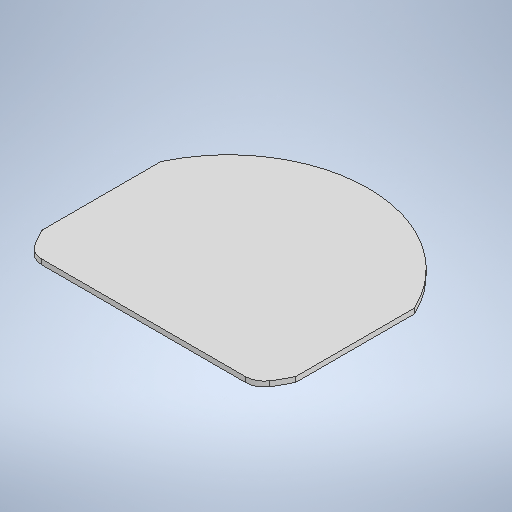
# Autodesk Inventor part: tapa_carcasa_4.0
Saved by Autodesk Inventor 2025.3 (Build 293356030, 356C)
## iProperties
Created: 2025-10-09
Part Number: tapa_carcasa_4.0
Material: Generic
Document SubType Name: Modeling
Designer: brene
Density: 1 g/cm^3
Appearance: Default
Author: brene
Autodesk Inventor part; units mm, degrees
ref_plane "YZ Plane" through (0, 0, 0) normal (1, 0, 0) x (0, 1, 0)
ref_plane "XZ Plane" through (0, 0, 0) normal (0, 1, 0) x (-1, 0, 0)
ref_plane "XY Plane" through (0, 0, 0) normal (0, 0, 1) x (1, 0, 0)
sketch "Sketch3" plane through (0, 0, 0) normal (0, 1, 0) x (-1, 0, 0)
  line L0 (0, 0) -> (67.5, 0)
  line L1 (0, 0) -> (0, 45)
  line L2 (67.5, 31.5278) -> (67.5, -31.5278)
  line L3 (0, 45) -> (54.1779, 45)
  line L4 (-67.5, 31.5278) -> (-67.5, -31.5278)
  line L5 (0, 45) -> (-54.1779, 45)
  arc A0 (67.5, 31.5278) -> (62.5776, 40.4264) centre (0, 0) ccw
  arc A1 (-62.5776, 40.4264) -> (-67.5, 31.5278) centre (0, 0) ccw
  arc A2 (-67.5, -31.5278) -> (67.5, -31.5278) centre (0, 0) ccw
  arc A3 (62.5776, 40.4264) -> (54.1779, 45) centre (54.1779, 35) ccw
  arc A4 (-54.1779, 45) -> (-62.5776, 40.4264) centre (-54.1779, 35) ccw
  point P0 (59.3738, 45)
  point P1 (-59.3738, 45)
  dimension "d28" = 67.5
  dimension "d29" = 45
  dimension "d30" = 10
  dimension "d31" = 10
  dimension "d32" = 74.5
  dimension "d34" = 67.5
  dimension "d35" = 74.5
  constraints: 12 end point, 12 point on circle, 5 centre point, 4 tangent, 3 symmetric about line, 2 horizontal, 2 point on line, 1 perpendicular, 1 vertical
  measures "d28" distance of L0.start L0.end
  measures "d29" distance of L0.start L1.end
  measures "d30" radius of A3
  measures "d31" radius of A4
  measures "d32" radius of A2
  measures "d34" distance between parallel lines of L2 L1
  measures "d35" radius of A1
extrude "Extrusion2" add sketch "Sketch3" along normal blind 2.7
body "Solid2"
